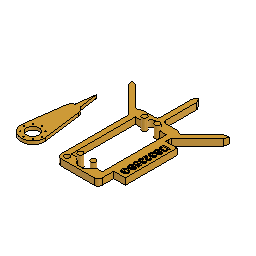
ds3235sg-servo-calibration-rig (Autodesk Fusion 360 design; units mm, degrees)
Autodesk Fusion 360 part; units mm, degrees
sketch "Sketch1" plane through (0, 0, 0) normal (0, 0, 1) x (1, 0, 0)
  line L0 (0, 0) -> (-32, 0)
  line L1 (-32, 0) -> (-32, -64)
  line L2 (-32, -64) -> (0, -64)
  line L3 (0, -64) -> (0, 0)
  line L4 (-4, -7.2) -> (-28, -7.2)
  line L5 (-28, -7.2) -> (-28, -56.8)
  line L6 (-28, -56.8) -> (-4, -56.8)
  line L7 (-4, -56.8) -> (-4, -7.2)
  line L8 (-4, -7.2) -> (-28, -56.8) construction
  line L9 (-28, -7.2) -> (-4, -56.8) construction
  line L10 (0, -32) -> (-32, -32) construction
  line L11 (-11.05, -61.8) -> (-20.95, -61.8)
  line L12 (-20.95, -61.8) -> (-20.95, -56.8)
  line L13 (-20.95, -56.8) -> (-11.05, -56.8)
  line L14 (-11.05, -56.8) -> (-11.05, -61.8)
  circle A0 centre (-11.05, -56.8) radius 2
  circle A1 centre (-20.95, -56.8) radius 2
  circle A2 centre (-11.05, -7.2) radius 2
  circle A3 centre (-20.95, -7.2) radius 2
  line L15 (-11.05, -2.2) -> (-20.95, -2.2)
  line L16 (-11.05, -7.2) -> (-11.05, -2.2)
  line L17 (-20.95, -2.2) -> (-20.95, -7.2)
  line L18 (-6, -52) -> (-26, -52)
  line L19 (-26, -52) -> (-26, -12)
  line L20 (-26, -12) -> (-6, -12)
  line L21 (-6, -12) -> (-6, -52)
  line L22 (-6, -52) -> (-26, -12) construction
  line L23 (-26, -52) -> (-6, -12) construction
  line L24 (-16, -12) -> (-16, -52) construction
  circle A4 centre (-16, -21.8) radius 4.75
  circle A5 centre (-16, -21.8) radius 9
  line L25 (-16, -21.8) -> (34, -21.8)
  line L26 (-16, -21.8) -> (19.3553, 13.5553)
  line L27 (-16, -21.8) -> (34, -21.8) construction
  line L28 (-14.4444, -23.0728) -> (20.6601, 12.0317)
  line L29 (-17.5556, -20.5272) -> (17.5867, 14.6152)
  line L30 (20.6601, 12.0317) -> (21.6436, 15.7022)
  line L31 (21.6436, 15.7022) -> (17.5867, 14.6152)
  line L32 (-14.4444, -20.5272) -> (-49.5867, 14.6152)
  line L33 (-16, -21.8) -> (-51.3553, 13.5553)
  line L34 (-17.5556, -23.0728) -> (-52.6601, 12.0317)
  line L35 (-52.6601, 12.0317) -> (-53.6436, 15.7022)
  line L36 (-53.6436, 15.7022) -> (-49.5867, 14.6152)
  line L37 (-16, -21.8) -> (-16, 28.2)
  line L38 (-14, -21.8) -> (-14, 28.2)
  line L39 (-18, -21.8) -> (-18, 28.2)
  line L40 (-14, 26.4489) -> (-16, 29.913)
  line L41 (-16, 29.913) -> (-18, 26.4489)
  line L42 (-6, -52) -> (9, -52)
  line L43 (9, -52) -> (9, -12)
  line L44 (9, -12) -> (-6, -12)
  line L45 (-6, -12) -> (-6, -52)
  line L46 (0.3217, -15.269) -> (0.3217, -42.8531) construction
  line L47 (0.3217, -42.8531) -> (6.8781, -42.8531) construction
  line L48 (6.8781, -42.8531) -> (6.8781, -15.269) construction
  line L49 (6.8781, -15.269) -> (0.3217, -15.269) construction
  circle A6 centre (-28, -60) radius 2
  circle A7 centre (-60.4284, -54.1396) radius 4.8
  circle A8 centre (-60.4284, -54.1396) radius 9
  line L50 (-60.4284, -54.1396) -> (-60.4284, -24.1396) construction
  circle A9 centre (-60.4284, -24.1396) radius 5
  line L51 (-65.3838, -23.4729) -> (-69.3481, -52.9396)
  line L52 (-55.4731, -23.4729) -> (-51.5088, -52.9396)
  line L53 (-60.5189, -4.1397) -> (-57.6827, -25.2216)
  line L54 (-60.338, -4.1397) -> (-63.1742, -25.2216)
  circle A10 centre (-60.4284, -54.1396) radius 7 construction
  circle A11 centre (-60.4284, -61.1396) radius 0.5
  circle A12 centre (-55.4787, -59.0894) radius 0.5
  circle A13 centre (-53.4284, -54.1396) radius 0.5
  circle A14 centre (-55.4787, -49.1899) radius 0.5
  circle A15 centre (-60.4284, -47.1396) radius 0.5
  circle A16 centre (-65.3782, -49.1899) radius 0.5
  circle A17 centre (-67.4284, -54.1396) radius 0.5
  circle A18 centre (-65.3782, -59.0894) radius 0.5
  point P0 (-16, -32)
  point P1 (-16, -32)
  point P2 (-16, -32)
  point P3 (-16, -21.8)
  point P4 (19.3553, 13.5553)
  point P5 (-16, 28.2)
  point P6 (-28, -60)
  point P7 (-60.5189, -4.1397)
  dimension "d1" = 32
  dimension "d2" = 64
  dimension "d3" = 49.6
  dimension "d4" = 24
  dimension "d5" = 9.9
  dimension "d6" = 5
  dimension "d7" = 4
  dimension "d12" = 20
  dimension "d13" = 40
  dimension "d14" = 9.8
  dimension "d15" = 9.5
  dimension "d16" = 18
  dimension "d17" = 50
  dimension "d18" = 45
  dimension "d19" = 50
  dimension "d28" = 50
  dimension "d29" = 2
  dimension "d30" = -2
  dimension "d35" = 15
  dimension "d36" = 40
  dimension "d37" = 5
  dimension "d42" = 4
  dimension "d43" = 4
  dimension "d44" = 4
  dimension "d52" = 9.6
  dimension "d53" = 18
  dimension "d54" = 10
  dimension "d55" = 30
  dimension "d56" = 50
  dimension "d59" = 14
  dimension "d60" = 1
  dimension "d62" = 360
  text T0 "DS3235SG" font "Arial" height 5 bold align left top in box 27.5841 x 6.5565 at (0.3217, -15.269) x (0, -1) y (1, 0) spacing 1 kerned
  constraint horizontal L0
  constraint vertical L1
  constraint horizontal L2
  constraint vertical L3
  constraint coincident L0.start L3.end
  constraint horizontal L4
  constraint perpendicular L4 L5
  constraint parallel L4 L6
  constraint parallel L5 L7
  constraint coincident L8 P2
  constraint coincident L9 P2
  constraint coincident P2 P1
  constraint midpoint L3 L10.start
  constraint midpoint L1 L10.end
  constraint midpoint P2 L10
  constraint horizontal L11
  constraint vertical L12
  constraint horizontal L13
  constraint vertical L14
  constraint midpoint L6 L13
  constraint coincident L13.end L14.start
  constraint coincident L12.end L13.start
  constraint equal A0 A1
  constraint symmetric L10 L11.start L15.start
  constraint symmetric L10 L11.end L15.end
  constraint symmetric L10 L12.end A3.centre
  constraint symmetric L10 L13.end A2.centre
  constraint symmetric L10 A0 A2
  constraint symmetric L10 A1 A3
  constraint horizontal L18
  constraint perpendicular L18 L19
  constraint parallel L18 L20
  constraint parallel L19 L21
  constraint coincident L22 P2
  constraint coincident L23 P2
  constraint midpoint L20 L24.start
  constraint midpoint L18 L24.end
  constraint coincident L24 P3
  constraint coincident P3 A4.centre
  constraint perpendicular L24 L25
  constraint horizontal L27
  constraint coincident P4 L26.end
  constraint symmetric L24 P3 A4.centre
  constraint symmetric L24 P4 L33.end
  constraint symmetric L24 L28.start L34.start
  constraint symmetric L24 L29.start L32.start
  constraint symmetric L24 L30.end L35.end
  constraint symmetric L24 L28.end L34.end
  constraint symmetric L24 L29.end L32.end
  constraint perpendicular L0 L37
  constraint coincident P5 L37.end
  constraint coincident L39 L41.end
  constraint coincident L38 L40.start
  constraint horizontal L42
  constraint vertical L43
  constraint horizontal L44
  constraint vertical L45
  constraint coincident P6 A6.centre
  constraint concentric A7 A8
  constraint coincident A7.centre A8.centre
  constraint vertical L50
  constraint coincident L50.end A9.centre
  constraint tangent A9 L51
  constraint tangent A8 L51
  constraint coincident A8 L51.end
  constraint coincident A9 L51.start
  constraint symmetric L50 L51.end L52.end
  constraint symmetric L50 L51.start L52.start
  constraint coincident P7 L53.start
  constraint parallel L52 L53
  constraint symmetric L50 P7 L54.start
  constraint symmetric L50 L53.end L54.end
  constraint concentric A8 A10
  constraint coincident A10 A11.centre
  measures "d1" distance of L0.start L0.end
  measures "d2" distance of L0.start L2.end
  measures "d3" distance of L4.end L5.end
  measures "d4" distance of L5.end L6.end
  measures "d5" distance of L11.start L11.end
  measures "d6" distance of L11.end L12.end
  measures "d7" diameter of A0
  measures "d12" distance of L19.end L20.end
  measures "d13" distance of L18.end L19.end
  measures "d14" distance of L24.start P3
  measures "d15" diameter of A4
  measures "d16" diameter of A5
  measures "d17" distance of P3 L25.end
  measures "d18" angle of L26 L27
  measures "d19" distance of P3 P4
  measures "d28" distance of P3 P5
  measures "d35" distance of L18.start L42.end
  measures "d36" distance of L18.start L20.end
  measures "d42" distance of L1 P6
  measures "d43" distance of L2 P6
  measures "d44" diameter of A6
  measures "d52" diameter of A7
  measures "d53" diameter of A8
  measures "d54" diameter of A9
  measures "d55" distance of A7.centre L50.end
  measures "d56" distance of A7.centre P7
  measures "d59" diameter of A10
  measures "d60" diameter of A11
extrude "Extrude1" add sketch "Sketch1" along normal blind 5 contours L0 L3 L4 A2 L15 L16 L29 L38 | L0 L15 L37 L38 | L3 L4 L7 L26 L29 | L0 L15 L37 L39 | L3 L7 L26 L28 L44 | L0 L1 L4 A3 L15 L17 L32 L39 | L3 L28 L44 | L3 L25 L43 L44 | L3 L7 L25 L28 L44 | L7 L28 L44 | L1 L4 L5 L32 L33 | L3 L25 L42 L43 | L3 L7 L25 L42 | L1 L5 L33 L34 | L1 L2 L3 L5 L6 L7 L11 L12 L14 A0 A1 L34 L42 | A6 makes body 1
extrude "Extrude2" add sketch "Sketch1" along normal blind 9 contours L4 A2 | L4 A2 L16 | L4 A2 L16 | L4 A3 L17 | L4 A3 L17 | L4 A3 | L6 L14 A0 | L6 L13 A0 | L6 L13 A1 | L6 L12 A1 | L6 L13 L14 A0 | L6 L12 L13 A1 bodies 1
extrude "Extrude3" add sketch "Sketch1" along normal blind 5 contours L0 L38 L39 L40 L41 | L3 L28 L29 L30 L31 | L1 L32 L34 L35 L36 bodies 1
extrude "Extrude5" cut sketch "Sketch1" along normal through all contours A6 bodies 1
fillet "Fillet1" radius 3 8 edges at (0, 0, 2.5) (-32, 0, 2.5) (-32, -64, 2.5) (0, -64, 2.5) (-20.95, -2.2, 2.5) (-11.05, -2.2, 2.5) (-20.95, -61.8, 2.5) (-11.05, -61.8, 2.5) on bodies 1
fillet "Fillet2" radius 2 4 edges at (-32, -8.6284, 2.5) (0, -8.6284, 2.5) (0, -2.9716, 2.5) (-32, -2.9716, 2.5) on bodies 1
fillet "Fillet2" radius 2 2 edges at (-18, 0, 2.5) (-14, 0, 2.5) on bodies 1
emboss "Emboss2" depth -2 profiles "Sketch1" section 1 text T0 onto face at (3, -38.6667, 5) on bodies 1 bodies 1
extrude "Extrude6" add sketch "Sketch1" along normal blind 2.5 separate body contours A8 | A8 A9 L51 L52 | A9 | A9 L53 L54 makes body 2
